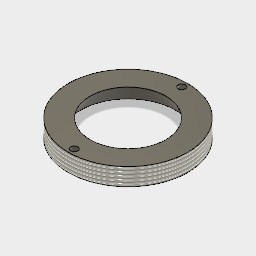
electrode punch tool cam v5 (Autodesk Fusion 360 archive; units mm, degrees)
design "Collet Top Taper"
Autodesk Fusion 360 part; units mm, degrees
sketch "Sketch1" plane through (0, 0, 0) normal (0, 0, 1) x (1, 0, 0)
  line L0 (-20.7744, 0) -> (-26.35, 0)
  line L1 (-26.35, 0) -> (-26.35, 7.62)
  line L2 (-26.35, 7.62) -> (-16.375, 7.62)
  line L3 (-16.375, 7.62) -> (-20.7744, 0)
  dimension "d1" = 26.35
  dimension "d2" = 16.375
  dimension "d3" = 60
  dimension "d4" = 7.62
  dimension "d5" = 7.62
  measures "d1" distance of origin L0.end
  measures "d2" distance of origin L2.end
  measures "d3" angle of L0 L3
  measures "d4" distance of L0.end L1.end
  measures "d5" distance of origin L2.end
sketch "Sketch2" plane through (0, 0, 0) normal (0, 0, 1) x (1, 0, 0)
  line L0 (0, 0) -> (0, 1)
  line L1 (0, 1) -> (0, 14) construction
revolve "Revolve1" add sketch "Sketch1" angle 360 about axis through (0, 1, 0) along (0, 1, 0)
thread "Thread1" "ISO Metric profile 52.0 M52x1.5 6g" major diameter 51.85 minor diameter 50.1269 pitch 1.5 angle 60 resizes the face on face at (-26.2191, 2.54, -2.6236)
sketch "Sketch3" plane through (0, 7.62, 0) normal (0, 1, 0) x (-1, 0, 0)
  circle A0 centre (0, 0) radius 25.925
  circle A1 centre (0, 0) radius 16.375
  point P0 (-0.0141, -23.35)
  point P1 (-0.0141, 23.35)
  dimension "d7" = 46.7
  dimension "d8" = 23.35
  measures "d7" distance of P0 P1
  measures "d8" distance of A0.centre P0
hole "Hole1" at (0.0141, 7.62, -23.35) at (0.0141, 7.62, 23.35) direction (0, -1, 0) diameter 3.1 depth 13.5 tip angle 118
equation "d1 = ( 52.7 / 2 ) * 1 mm"
equation "d2 = ( 32.75 / 2 ) * 1 mm"

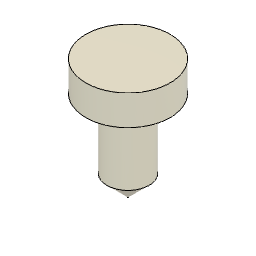
design "electrode punch tool"
Autodesk Fusion 360 part; units mm, degrees
sketch "Sketch1" plane through (0, 0, 0) normal (0, 0, 1) x (1, 0, 0)
  line L0 (0, 0) -> (3.5, 3.5)
  line L1 (3.5, 3.5) -> (3.5, 15)
  line L2 (3.5, 15) -> (11, 15)
  line L3 (11, 15) -> (11, 20)
  line L4 (11, 20) -> (0, 20)
  line L5 (0, 20) -> (0, 0)
  line L6 (0.025, 0.025) -> (0, 0.025)
  line L7 (3.5, 3.5) -> (11, 3.5)
  line L8 (11, 3.5) -> (11, 15)
  line L9 (12.5, 4.5) -> (12.5, -5.5)
  line L10 (12.5, -5.5) -> (0, -5.5)
  line L11 (0, -5.5) -> (0, 0)
  line L12 (12.5, 4.5) -> (11, 4.5)
  line L13 (3.5, 3.5) -> (3.5, -5.5)
  dimension "d1" = 45
  dimension "d2" = 3.5
  dimension "d3" = 15
  dimension "d4" = 5
  dimension "d5" = 11
  dimension "d7" = 0.025
  dimension "d8" = 12.5
  dimension "d9" = 1
  dimension "d10" = 10
  constraint coincident L0.start L5.end
  constraint vertical L1
  constraint perpendicular L1 L2
  constraint perpendicular L2 L3
  constraint perpendicular L3 L4
  constraint perpendicular L4 L5
  constraint coincident L0 L6.start
  constraint coincident L5 L6.end
  constraint perpendicular L5 L6
  constraint perpendicular L1 L7
  constraint vertical L8
  constraint vertical L9
  constraint perpendicular L9 L10
  constraint perpendicular L10 L11
  constraint coincident L8 L12.end
  constraint perpendicular L8 L12
  constraint coincident L10 L13.end
  constraint perpendicular L10 L13
  measures "d1" angle of L0 L5
  measures "d2" distance of L1 L5
  measures "d3" distance of L0.start L2
  measures "d4" distance of L2.end L3.end
  measures "d5" distance of L3.end L4.end
  measures "d7" distance of L6.start L6.end
  measures "d8" distance of L9.end L10.end
  measures "d9" distance of L7 L12
  measures "d10" distance of L9.start L9.end
revolve "Revolve1" add sketch "Sketch1" angle 360 about axis through (0, 20, 0) along (0, -1, 0) contours L0 L1 L2 L3 L4 L5 L6 makes body 1
revolve "Revolve2" add sketch "Sketch1" angle 360 about axis through (0, 3.5, 0) along (0, 1, 0) separate body contours L1 L2 L7 L8 makes body 2
revolve "Revolve3" add sketch "Sketch1" angle 360 about axis through (0, 3.5, 0) along (0, 1, 0) separate body contours L7 L8 L9 L10 L12 L13 makes body 3
move_face "OffsetFaces1" offset -0.1 1 faces at (3.4826, 11.1667, 0.3485) on bodies 2
move_face "OffsetFaces2" offset -0.3 1 faces at (3.4826, -2.5, 0.3485) on bodies 3
move_face "OffsetFaces3" offset -0.3 1 faces at (10.9453, 4.1667, 1.0952) on bodies 3
move_face "OffsetFaces4" offset -4 1 faces at (10.9863, 16.6667, -0.5483) on bodies 1
copy_body "Body->Comp1" bodies 1 removing the originals makes body 4 in component "punch"
copy_body "Body->Comp2" bodies 2 removing the originals makes body 5 in component "guide"
copy_body "Body->Comp3" bodies 3 removing the originals makes body 6 in component "die"
component "punch" placed x (1, 0, 0) y (0, 1, 0) z (0, 0, 1) at (0, 0, 0)
component "guide" placed x (1, 0, 0) y (0, 1, 0) z (0, 0, 1) at (0, 0, 0)
component "die" placed x (1, 0, 0) y (0, 1, 0) z (0, 0, 1) at (0, 0, 0)
named bodies: "punch", "guide", "die"

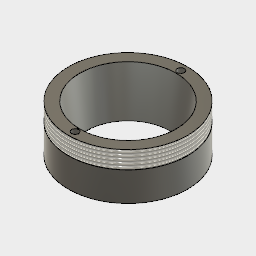
design "Collet Bottom Taper"
Autodesk Fusion 360 part; units mm, degrees
sketch "Sketch1" plane through (0, 0, 0) normal (0, 0, 1) x (1, 0, 0)
  line L0 (-18.15, 0) -> (-25.95, 0)
  line L1 (-25.95, 0) -> (-25.95, 12.7)
  line L2 (-25.95, 12.7) -> (-26.375, 12.7)
  line L3 (-26.375, 12.7) -> (-26.375, 20.32)
  line L4 (-26.375, 20.32) -> (-21.0058, 20.32)
  line L5 (-21.0058, 20.32) -> (-18.15, 0)
  dimension "d1" = 25.95
  dimension "d2" = 26.375
  dimension "d3" = 12.7
  dimension "d4" = 7.62
  dimension "d5" = 98
  dimension "d6" = 7.8
  dimension "d7" = 20.32
  measures "d1" distance of origin L1
  measures "d2" distance of origin L3
  measures "d3" distance of L0.end L1.end
  measures "d4" distance of L2.end L3.end
  measures "d5" angle of L0 L5
  measures "d6" distance of L0.end L0.start
  measures "d7" distance of origin L4.end
sketch "Sketch2" plane through (0, 0, 0) normal (0, 0, 1) x (1, 0, 0)
  line L0 (-18.15, 0) -> (-25.95, 0)
  line L1 (0, 0) -> (0, 22) construction
revolve "Revolve1" add sketch "Sketch1" angle 360 about axis through (0, 0, 0) along (0, 1, 0)
thread "Thread1" "ISO Metric profile 52.0 M52x1.5 6g" major diameter 51.85 minor diameter 50.1269 pitch 1.5 angle 60 resizes the face on face at (-26.3422, 15.24, -1.3147)
sketch "Sketch3" plane through (0, 20.32, 0) normal (0, 1, 0) x (-1, 0, 0)
  circle A0 centre (0, 0) radius 25.925
  circle A1 centre (0, 0) radius 21.0058
  point P0 (0, -23)
  point P1 (0, 23)
  dimension "d9" = 46
  dimension "d10" = 23
  measures "d9" distance of P0 P1
  measures "d10" distance of A0.centre P0
hole "Hole1" at (0, 20.32, -23) at (0, 20.32, 23) direction (0, -1, 0) diameter 3.1 depth 13.5 tip angle 118
equation "d1 = ( 51.9 / 2 ) * 1 mm"
equation "d2 = ( 52.75 / 2 ) * 1 mm"
